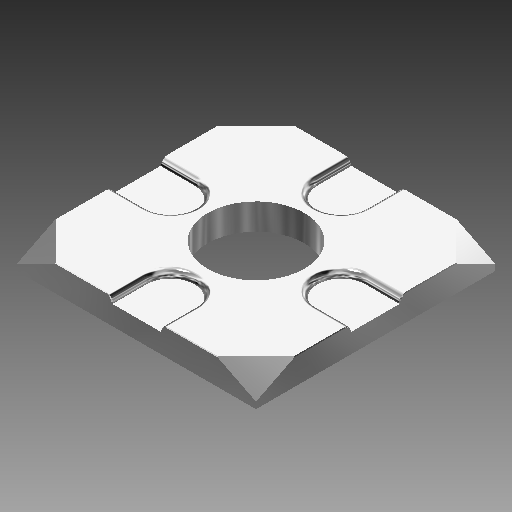
# Autodesk Inventor part: SSR-40 DA Small Plate
Saved by Autodesk Inventor 2019 (Build 230136000, 136)
## iProperties
Created: 2014-10-31
Part Number: SSR-40 DA Small Plate
Material: Nickel-Copper Alloy 400
Document SubType Name: Modeling
Designer: Tyler
Density: 8.83 g/cm^3
Appearance: Chrome - Polished
Mass: 0.719434 g
Surface Area: 2.16818 cm^2
Volume: 0.0814761 cm^3
Author: Tyler
Autodesk Inventor part; units mm, degrees
ref_plane "YZ Plane" through (0, 0, 0) normal (1, 0, 0) x (0, 1, 0)
ref_plane "XZ Plane" through (0, 0, 0) normal (0, 1, 0) x (-1, 0, 0)
ref_plane "XY Plane" through (0, 0, 0) normal (0, 0, 1) x (1, 0, 0)
sketch "Sketch1" plane through (0, 0, 0) normal (0, 1, 0) x (-1, 0, 0)
  line L0 (4.8641, 4.8641) -> (-4.8641, 4.8641)
  line L1 (-4.8641, 4.8641) -> (-4.8641, -4.8641)
  line L2 (-4.8641, -4.8641) -> (4.8641, -4.8641)
  line L3 (4.8641, -4.8641) -> (4.8641, 4.8641)
  point P0 (0, 0)
  point P1 (4.8641, 0)
  point P2 (0, -4.8641)
  dimension "d0" = 9.7282
  dimension "d1" = 9.7282
  constraints: 8 end point, 2 midpoint, 2 parallel, 1 horizontal, 1 horizontal alignment, 1 perpendicular, 1 vertical alignment
  measures "d0" distance of L2.end L1.end
  measures "d1" distance of L1.end L0.end
extrude "Extrusion1" add sketch "Sketch1" along normal blind 1.0668
sketch "Sketch2" plane through (0, 1.0668, 0) normal (0, 1, 0) x (1, 0, 0)
  line L0 (-4.8641, -4.8641) -> (4.8641, -4.8641) projected
  line L1 (3.4798, -0.9779) -> (4.8641, -0.9779)
  line L2 (4.8641, -0.9779) -> (4.8641, 0.9779)
  line L3 (4.8641, 0.9779) -> (3.4798, 0.9779)
  line L4 (2.5019, 0) -> (2.5019, 0)
  arc A0 (2.5019, 0) -> (3.4798, -0.9779) centre (3.4798, 0) ccw
  arc A1 (3.4798, 0.9779) -> (2.5019, 0) centre (3.4798, 0) ccw
  line L5 (4.8641, -4.8641) -> (4.8641, 4.8641) projected
  line L6 (0, 2.5019) -> (0, 2.5019)
  line L7 (-0.9779, 3.4798) -> (-0.9779, 4.8641)
  line L8 (-0.9779, 4.8641) -> (0.9779, 4.8641)
  line L9 (0.9779, 4.8641) -> (0.9779, 3.4798)
  arc A2 (0, 2.5019) -> (0.9779, 3.4798) centre (0, 3.4798) ccw
  arc A3 (-0.9779, 3.4798) -> (0, 2.5019) centre (0, 3.4798) ccw
  line L10 (4.8641, 4.8641) -> (-4.8641, 4.8641) projected
  line L11 (-4.8641, -0.9779) -> (-3.4798, -0.9779)
  line L12 (-2.5019, 0) -> (-2.5019, 0)
  line L13 (-3.4798, 0.9779) -> (-4.8641, 0.9779)
  line L14 (-4.8641, 0.9779) -> (-4.8641, -0.9779)
  line L15 (-4.8641, 4.8641) -> (-4.8641, -4.8641) projected
  arc A4 (-3.4798, -0.9779) -> (-2.5019, 0) centre (-3.4798, 0) ccw
  arc A5 (-2.5019, 0) -> (-3.4798, 0.9779) centre (-3.4798, 0) ccw
  line L16 (-0.9779, -4.8641) -> (0.9779, -4.8641)
  line L17 (0.9779, -4.8641) -> (0.9779, -3.4798)
  line L18 (0, -2.5019) -> (0, -2.5019)
  line L19 (-0.9779, -3.4798) -> (-0.9779, -4.8641)
  arc A6 (0, -2.5019) -> (-0.9779, -3.4798) centre (0, -3.4798) ccw
  arc A7 (0.9779, -3.4798) -> (0, -2.5019) centre (0, -3.4798) ccw
  point P0 (0, 0)
  point P1 (4.8641, 0)
  point P2 (4.8641, 0)
  point P3 (0, -4.8641)
  point P4 (0, -4.8641)
  point P5 (0, -4.8641)
  point P6 (-0.9779, 2.5019)
  point P7 (0, 4.8641)
  point P8 (0, 4.8641)
  point P9 (-2.5019, 0.9779)
  point P10 (-4.8641, 0)
  point P11 (-4.8641, 0)
  point P12 (0.9779, -2.5019)
  point P13 (0, -4.8641)
  point P14 (0, -4.8641)
  dimension "d10" = 0.9779
  dimension "d11" = 1.9558
  dimension "d12" = 2.3622
  dimension "d13" = 2.3622
  dimension "d14" = 0.9779
  dimension "d15" = 2.3622
  dimension "d16" = 0.9779
  dimension "d17" = 2.3622
  dimension "d18" = 0.9779
  constraints: 32 end point, 16 point on circle, 16 tangent, 10 midpoint, 8 centre point, 8 parallel, 6 point on line, 4 coincident, 4 concentric, 4 horizontal, 4 perpendicular, 2 horizontal alignment, 2 vertical alignment
  measures "d10" radius of A0
  measures "d11" distance of L1.end L2.end
  measures "d12" distance from line of L2 L4.end
  measures "d13" distance of point (-0.978, 2.502) L7.end
  measures "d14" radius of A2
  measures "d15" distance of L13.end point (-2.502, 0.978)
  measures "d16" radius of A4
  measures "d17" distance of point (0.978, -2.502) L16.end
  measures "d18" radius of A6
extrude "Extrusion2" cut sketch "Sketch2" against normal blind 0.2794 contours L19 A6 A7 L17 L0 | L14 L13 A5 A4 L11 | L1 A0 A1 L3 L2 | L8 L9 A2 A3 L7
fillet "Fillet1" radius 0.2794 12 edges at (0, 1.0668, 2.5019) (0.9779, 1.0668, 4.1719) (-0.9779, 1.0668, 4.1719) (-4.1719, 1.0668, 0.9779) (-4.1719, 1.0668, -0.9779) (-2.5019, 1.0668, 0) (-0.9779, 1.0668, -4.172) (0.9779, 1.0668, -4.172) (0, 1.0668, -2.5019) (4.172, 1.0668, -0.9779) (4.172, 1.0668, 0.9779) (2.5019, 1.0668, 0)
sketch "Sketch3" plane through (0, 1.0668, 0) normal (0, 1, 0) x (1, 0, 0)
  circle A0 centre (0, 0) radius 1.9685
  dimension "d22" = 3.937
  constraints: 1 centre point, 1 coincident
  measures "d22" diameter of A0
extrude "Extrusion3" cut sketch "Sketch3" against normal through all
chamfer "Chamfer1" distance 0.0254 angle 45 16 edges at (3.0605, 1.0668, 4.8641) (1.0596, 0.9851, 4.8641) (4.8641, 1.0668, 3.0604) (4.8641, 0.9851, 1.0596) (4.8641, 1.0668, -3.0605) (4.8641, 0.9851, -1.0596) (3.0605, 1.0668, -4.8641) (1.0596, 0.9851, -4.8641) (-3.0605, 1.0668, -4.8641) (-1.0596, 0.9851, -4.8641) (-4.8641, 1.0668, -3.0605) (-4.8641, 0.9851, -1.0596) (-4.8641, 1.0668, 3.0605) (-4.8641, 0.9851, 1.0596) (-3.0605, 1.0668, 4.8641) (-1.0596, 0.9851, 4.8641)
chamfer "Chamfer2" distance 1.27 angle 45 4 edges at (4.8514, 1.0541, 4.8514) (4.8514, 1.0541, -4.8514) (-4.8514, 1.0541, -4.8514) (-4.8514, 1.0541, 4.8514)
body "Solid1"
